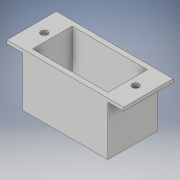
# Autodesk Inventor part: servopocket
Saved by Autodesk Inventor 2018 (Build 220112000, 112)
## iProperties
Created: 2017-12-28
Part Number: servopocket
Material: Generic
Document SubType Name: Modeling
Designer: BB-8
Density: 1 g/cm^3
Appearance: Default
Author: BB-8
Autodesk Inventor part; units mm, degrees
ref_plane "YZ Plane" through (0, 0, 0) normal (1, 0, 0) x (0, 1, 0)
ref_plane "XZ Plane" through (0, 0, 0) normal (0, 1, 0) x (-1, 0, 0)
ref_plane "XY Plane" through (0, 0, 0) normal (0, 0, 1) x (1, 0, 0)
sketch "Sketch1" plane through (0, 0, 0) normal (0, 1, 0) x (-1, 0, 0)
  point P0 (0, 0)
sketch "Sketch2" plane through (0, 0, 0) normal (0, 1, 0) x (-1, 0, 0)
  line L0 (0, 0) -> (22.5, 0)
  line L1 (22.5, 0) -> (22.5, -11.8)
  line L2 (22.5, -11.8) -> (0, -11.8)
  line L3 (0, -11.8) -> (0, 0)
  line L4 (24, -13.3) -> (24, 1.5)
  line L5 (24, 1.5) -> (-1.5, 1.5)
  line L6 (-1.5, 1.5) -> (-1.5, -13.3)
  line L7 (-1.5, -13.3) -> (24, -13.3)
  dimension "d0" = 22.5
  dimension "d1" = 11.8
  dimension "d2" = 1.5
  constraints: 16 end point, 4 parallel, 2 perpendicular, 1 horizontal, 3 other
  measures "d0" distance of L1.end L2.end
  measures "d1" distance of L0.end L1.end
  measures "d2" distance between parallel lines of L1 L4
extrude "Extrusion1" add sketch "Sketch2" along normal blind 15.9
sketch "Sketch3" plane through (0, 15.9, 0) normal (0, 1, 0) x (1, 0, 0)
  line L0 (-24, -1.5) -> (1.5, -1.5) projected
  line L1 (1.5, -1.5) -> (6.2, -1.5)
  line L2 (6.2, -1.5) -> (6.2, 13.3)
  line L3 (6.2, 13.3) -> (1.5, 13.3)
  line L4 (1.5, 13.3) -> (1.5, -1.5)
  line L5 (-24, 13.3) -> (-24, -1.5) projected
  line L6 (-24, -1.5) -> (-28.7, -1.5)
  line L7 (-28.7, -1.5) -> (-28.7, 13.3)
  line L8 (-28.7, 13.3) -> (-24, 13.3)
  line L9 (-24, 13.3) -> (-24, -1.5)
  point P0 (0, 0)
  dimension "d5" = 4.7
  dimension "d6" = 4.7
  constraints: 16 end point, 4 parallel, 2 horizontal, 2 perpendicular
  measures "d5" distance of L3.end L2.end
  measures "d6" distance of L7.end L8.end
extrude "Extrusion2" add sketch "Sketch3" against normal blind 1
sketch "Sketch4" plane through (0, 15.9, 0) normal (0, 1, 0) x (1, 0, 0)
  line L0 (0, 11.8) -> (0, 0) projected
  line L1 (0, 5.9) -> (2.4, 5.9)
  circle A0 centre (2.4, 5.9) radius 1
  line L2 (-28.7, -1.5) -> (6.2, -1.5) projected
  line L3 (-11.25, -1.5) -> (-11.25, 13.3)
  line L4 (6.2, 13.3) -> (-28.7, 13.3) projected
  circle A1 centre (-24.9, 5.9) radius 1
  dimension "d9" = 2.4
  dimension "d10" = 2
  constraints: 4 end point, 3 midpoint, 2 centre point, 1 coincident, 1 horizontal, 1 symmetric about line, 1 other
  measures "d9" distance of L1.start L1.end
  measures "d10" diameter of A0
extrude "Extrusion3" cut sketch "Sketch4" against normal blind 2
body "Solid1"
